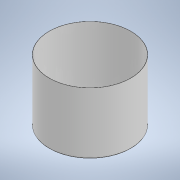
# Autodesk Inventor part: distilate_tank
Saved by Autodesk Inventor 2020 (Build 240168000, 168)
## iProperties
Created: 2022-09-01
Part Number: distilate_tank
Material: Generic
Document SubType Name: Modeling
Designer: Intuito_PC
Density: 1 g/cm^3
Appearance: Default
Author: Intuito_PC
Autodesk Inventor part; units mm, degrees
ref_plane "YZ Plane" through (0, 0, 0) normal (1, 0, 0) x (0, 1, 0)
ref_plane "XZ Plane" through (0, 0, 0) normal (0, 1, 0) x (-1, 0, 0)
ref_plane "XY Plane" through (0, 0, 0) normal (0, 0, 1) x (1, 0, 0)
sketch "Sketch1" plane through (0, 0, 0) normal (0, 1, 0) x (-1, 0, 0)
  circle A0 centre (0, 0) radius 200
  dimension "d0" = 400
  constraints: 1 centre point, 1 coincident
  measures "d0" diameter of A0
extrude "Extrusion1" add sketch "Sketch1" along normal blind 300
shell "Shell1" thickness 1 removed faces 1 at (26.6799, 300, 17.8469)
fillet "Fillet1" radius 3.175 1 edges at (200, 0, 0)
body "Solid1"
